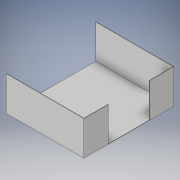
# Autodesk Inventor part: hopper_bottom2
Saved by Autodesk Inventor 2017 (Build 210142000, 142)
## iProperties
Created: 2020-02-21
Part Number: hopper_bottom2
Material: Generic
Document SubType Name: Modeling
Designer: S338674153
Density: 1 g/cm^3
Appearance: Default
Author: S338674153
Autodesk Inventor part; units mm, degrees
ref_plane "YZ Plane" through (0, 0, 0) normal (1, 0, 0) x (0, 1, 0)
ref_plane "XZ Plane" through (0, 0, 0) normal (0, 1, 0) x (-1, 0, 0)
ref_plane "XY Plane" through (0, 0, 0) normal (0, 0, 1) x (1, 0, 0)
sketch "Sketch1" plane through (0, 0, 0) normal (0, 1, 0) x (-1, 0, 0)
  line L0 (0, 0) -> (406.4, 0)
  line L1 (406.4, 0) -> (406.4, -469.9)
  line L2 (406.4, -469.9) -> (0, -469.9)
  line L3 (0, -469.9) -> (0, 0)
  dimension "d0" = 406.4
  dimension "d1" = 469.9
  constraints: 8 end point, 2 parallel, 1 horizontal, 1 perpendicular
  measures "d0" distance of L1.end L2.end
  measures "d1" distance of L0.end L1.end
extrude "Extrusion1" add sketch "Sketch1" along normal blind 1.905
sketch "Sketch2" plane through (0, 1.905, 0) normal (0, 1, 0) x (1, 0, 0)
  line L0 (-406.4, 469.9) -> (-406.4, 0) projected
  line L1 (0, 0) -> (0, 469.9) projected
  line L2 (-406.4, 0) -> (0, 0)
  line L3 (0, 0) -> (0, 1.905)
  line L4 (-1.905, 1.905) -> (-406.4, 1.905)
  line L5 (-406.4, 1.905) -> (-406.4, 0)
  line L6 (0, 469.9) -> (-406.4, 469.9) projected
  line L7 (0, 0) -> (-52.705, 0)
  line L8 (-1.905, 1.905) -> (-1.905, 467.995)
  line L9 (-1.905, 469.9) -> (0, 469.9)
  line L10 (0, 469.9) -> (0, 0)
  line L11 (0, 469.9) -> (-406.4, 469.9)
  line L12 (-406.4, 469.9) -> (-406.4, 467.995)
  line L13 (-406.4, 467.995) -> (-1.905, 467.995)
  line L14 (0, 467.995) -> (0, 469.9)
  dimension "d4" = 1.905
  dimension "d5" = 1.905
  dimension "d6" = 1.905
  dimension "d13" = 1.905
  constraints: 24 end point, 6 parallel, 3 horizontal, 3 perpendicular, 3 point on line
  measures "d4" distance of L3.end L2.end
  measures "d5" distance of L9.start L9.end
  measures "d6" distance of L12.end L11.end
  measures "d13" distance between parallel lines of L10 L8
extrude "Extrusion2" add sketch "Sketch2" along normal blind 177.8 contours L6 L1 L2 L0 L4 L8 L13
sketch "Sketch3" plane through (0, 179.705, 0) normal (0, 1, 0) x (1, 0, 0)
  line L0 (-1.905, 467.995) -> (-1.905, 1.905) projected
  line L1 (0, 469.9) -> (0, 0) projected
  line L2 (-1.905, 342.9) -> (0, 342.9)
  line L3 (0, 342.9) -> (0, 127)
  line L4 (0, 127) -> (-1.905, 127)
  line L5 (-1.905, 127) -> (-1.905, 342.9)
  line L6 (-406.4, 0) -> (0, 0) projected
  line L7 (0, 469.9) -> (-406.4, 469.9) projected
  dimension "d9" = 127
  dimension "d10" = 127
  constraints: 8 end point, 2 parallel, 2 point on line, 1 horizontal, 1 perpendicular
  measures "d9" distance between parallel lines of L6 L4
  measures "d10" distance between parallel lines of L7 L2
extrude "Extrusion3" cut sketch "Sketch3" against normal blind 177.8
body "Solid1"
